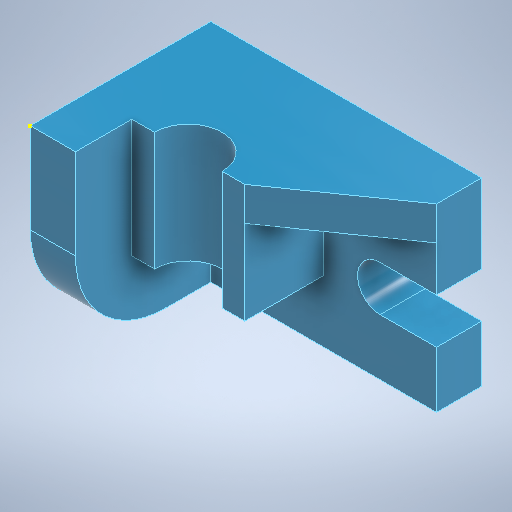
# Autodesk Inventor part: exercise
Saved by Autodesk Inventor 2025.1 (Build 291241000, 241)
## iProperties
Created: 2024-10-23
Part Number: exercise
Material: Generic
Document SubType Name: Modeling
Designer: kamil
Density: 1 g/cm^3
Appearance: Sky Blue Dark
Author: kamil
Autodesk Inventor part; units mm, degrees
ref_plane "YZ Plane" through (0, 0, 0) normal (1, 0, 0) x (0, 1, 0)
ref_plane "XZ Plane" through (0, 0, 0) normal (0, 1, 0) x (-1, 0, 0)
ref_plane "XY Plane" through (0, 0, 0) normal (0, 0, 1) x (1, 0, 0)
sketch "Sketch1" plane through (0, 0, 0) normal (0, 0, 1) x (1, 0, 0)
  line L0 (0, 0) -> (96, 0)
  line L1 (96, 0) -> (96, -64)
  line L2 (96, -64) -> (0, -64)
  line L3 (0, -64) -> (0, 0)
  dimension "d0" = 96
  constraints: 8 end point, 2 parallel, 1 horizontal, 1 perpendicular
  measures "d0" distance of L1.end L2.end
extrude "Extrusion1" add sketch "Sketch1" along normal blind 16
sketch "Sketch2" plane through (0, 0, 16) normal (0, 0, 1) x (1, 0, 0)
  line L0 (0, 0) -> (16, 0)
  line L1 (16, 0) -> (16, -64)
  line L2 (16, -64) -> (0, -64)
  line L3 (0, -64) -> (0, 0)
  line L4 (0, -64) -> (96, -64) projected
  dimension "d4" = 16
  constraints: 8 end point, 2 parallel, 1 collinear, 1 horizontal, 1 perpendicular
  measures "d4" distance of L1.end L2.end
extrude "Extrusion2" add sketch "Sketch2" along normal blind 48
sketch "Sketch3" plane through (0, 0, 64) normal (0, 0, 1) x (1, 0, 0)
  point P0 (0, 0)
fillet "Fillet1" radius 32 1 edges at (8, -64, 64)
sketch "Sketch4" plane through (0, 0, 0) normal (0, 1, 0) x (1, 0, 0)
  line L0 (16, -16) -> (96, -16) projected
  line L1 (16, -16) -> (56, -16)
  line L2 (56, -16) -> (56, -44)
  line L3 (16, -44) -> (16, -16)
  arc A0 (48, -44) -> (24, -44) centre (36, -44) ccw
  line L4 (56, -44) -> (48, -44)
  line L5 (24, -44) -> (16, -44)
  point P0 (0, 0)
  dimension "d8" = 40
  dimension "d9" = 28
  dimension "d10" = 24
  constraints: 10 end point, 3 parallel, 2 point on circle, 1 centre point, 1 horizontal, 1 perpendicular
  measures "d8" distance of L2.end L3.start
  measures "d9" distance of L1.end L2.end
  measures "d10" diameter of A0
extrude "Extrusion3" add sketch "Sketch4" against normal blind 42
sketch "Sketch5" plane through (0, 0, 0) normal (0, 1, 0) x (1, 0, 0)
  line L0 (16, -16) -> (96, -16) projected
  line L1 (56, -44) -> (48, -44) projected
  line L2 (96, -16) -> (56, -44)
  line L3 (56, -16) -> (56, -44) projected
  line L4 (56, -44) -> (56, -16)
  line L5 (56, -16) -> (96, -16)
  point P0 (0, 0)
  constraints: 6 end point, 1 collinear, 1 perpendicular
extrude "Extrusion4" add sketch "Sketch5" against normal blind 12
sketch "Sketch6" plane through (0, 0, 16) normal (0, 0, 1) x (1, 0, 0)
  line L0 (96, -64) -> (96, -12) projected
  line L1 (96, -44) -> (76, -44)
  arc A0 (76, -28) -> (76, -44) centre (76, -36) ccw
  line L2 (76, -28) -> (96, -28)
  line L3 (96, -28) -> (96, -44)
  point P0 (0, 0)
  dimension "d15" = 20
  dimension "d16" = 52
  dimension "d17" = 16
  dimension "d18" = 32
  constraints: 6 end point, 3 perpendicular, 2 point on circle, 2 point on line, 1 centre point, 1 tangent
  measures "d15" distance of L1.start L1.end
  measures "d16" distance of L0.start L0.end
  measures "d17" distance of L0.end L2.end
  measures "d18" distance of L0.end L1.start
extrude "Extrusion5" cut sketch "Sketch6" against normal blind 16
body "Solid1"
